Autodesk Fusion 360 part; units mm, degrees
(part 20 of 25)
sketch "Top Component Outlines" plane through (0, 0, 0) normal (0, 0, 1) x (1, 0, 0)
  arc A0 (71.501, 48.2981) -> (71.501, 48.2219) centre (71.501, 48.26) ccw
  arc A1 (71.501, 48.2219) -> (71.501, 48.2981) centre (71.501, 48.26) ccw
  arc A2 (76.0349, 48.514) -> (76.1111, 48.514) centre (76.073, 48.514) ccw
  arc A3 (73.9775, 50.292) -> (73.8505, 50.292) centre (73.914, 50.292) ccw
  arc A4 (75.819, 48.2219) -> (75.819, 48.2981) centre (75.819, 48.26) ccw
  arc A5 (73.9775, 49.53) -> (73.8505, 49.53) centre (73.914, 49.53) ccw
  arc A6 (71.501, 50.8) -> (71.247, 50.546) centre (71.501, 50.546) ccw
  arc A7 (76.1111, 50.546) -> (76.0349, 50.546) centre (76.073, 50.546) ccw
  arc A8 (71.501, 50.7619) -> (71.501, 50.8381) centre (71.501, 50.8) ccw
  arc A9 (73.3425, 49.53) -> (73.4695, 49.53) centre (73.406, 49.53) ccw
  arc A10 (71.501, 50.8381) -> (71.501, 50.7619) centre (71.501, 50.8) ccw
  arc A11 (71.2851, 48.514) -> (71.2089, 48.514) centre (71.247, 48.514) ccw
  arc A12 (73.3425, 48.768) -> (73.4695, 48.768) centre (73.406, 48.768) ccw
  line L0 (74.041, 49.53) -> (73.914, 49.53)
  line L1 (71.247, 50.546) -> (71.247, 48.514)
  arc A13 (71.2089, 48.514) -> (71.2851, 48.514) centre (71.247, 48.514) ccw
  line L2 (71.501, 50.8) -> (75.819, 50.8)
  arc A14 (76.0349, 50.546) -> (76.1111, 50.546) centre (76.073, 50.546) ccw
  arc A15 (76.1111, 48.514) -> (76.0349, 48.514) centre (76.073, 48.514) ccw
  arc A16 (71.2089, 50.546) -> (71.2851, 50.546) centre (71.247, 50.546) ccw
  line L3 (73.914, 49.53) -> (73.914, 48.768)
  line L4 (75.819, 48.26) -> (71.501, 48.26)
  arc A17 (71.247, 48.514) -> (71.501, 48.26) centre (71.501, 48.514) ccw
  arc A18 (73.4695, 50.292) -> (73.3425, 50.292) centre (73.406, 50.292) ccw
  arc A19 (75.819, 50.8381) -> (75.819, 50.7619) centre (75.819, 50.8) ccw
  arc A20 (73.914, 49.5681) -> (73.914, 49.4919) centre (73.914, 49.53) ccw
  arc A21 (74.041, 49.4919) -> (74.041, 49.5681) centre (74.041, 49.53) ccw
  arc A22 (76.073, 50.546) -> (75.819, 50.8) centre (75.819, 50.546) ccw
  arc A23 (75.819, 50.7619) -> (75.819, 50.8381) centre (75.819, 50.8) ccw
  arc A24 (71.2851, 50.546) -> (71.2089, 50.546) centre (71.247, 50.546) ccw
  arc A25 (75.819, 48.26) -> (76.073, 48.514) centre (75.819, 48.514) ccw
  arc A26 (75.819, 48.2981) -> (75.819, 48.2219) centre (75.819, 48.26) ccw
  line L5 (73.406, 49.53) -> (73.279, 49.53)
  arc A27 (73.406, 49.4919) -> (73.406, 49.5681) centre (73.406, 49.53) ccw
  arc A28 (73.8505, 49.53) -> (73.9775, 49.53) centre (73.914, 49.53) ccw
  arc A29 (73.4695, 49.53) -> (73.3425, 49.53) centre (73.406, 49.53) ccw
  arc A30 (73.279, 49.5681) -> (73.279, 49.4919) centre (73.279, 49.53) ccw
  line L6 (76.073, 50.546) -> (76.073, 48.514)
  arc A31 (73.8505, 48.768) -> (73.9775, 48.768) centre (73.914, 48.768) ccw
  line L7 (73.914, 49.53) -> (73.914, 50.292)
  line L8 (73.406, 50.292) -> (73.406, 49.53)
  line L9 (73.406, 49.53) -> (73.406, 48.768)
  arc A32 (14.605, 38.9509) -> (14.605, 39.0271) centre (14.605, 38.989) ccw
  line L10 (12.7, 37.338) -> (15.24, 37.338)
  line L11 (15.24, 37.338) -> (15.24, 37.846)
  line L12 (13.97, 38.989) -> (14.605, 38.989)
  arc A33 (13.97, 39.0271) -> (13.97, 38.9509) centre (13.97, 38.989) ccw
  arc A34 (15.2019, 36.957) -> (15.2781, 36.957) centre (15.24, 36.957) ccw
  arc A35 (50.3809, 18.669) -> (50.4571, 18.669) centre (50.419, 18.669) ccw
  line L13 (13.97, 38.354) -> (13.97, 38.989)
  arc A36 (14.605, 39.9669) -> (14.605, 40.0431) centre (14.605, 40.005) ccw
  line L14 (14.351, 41.021) -> (14.351, 42.926)
  arc A37 (50.4571, 19.05) -> (50.3809, 19.05) centre (50.419, 19.05) ccw
  arc A38 (52.07, 20.574) -> (52.07, 14.986) centre (52.07, 17.78) ccw
  arc A39 (15.2781, 41.021) -> (15.2019, 41.021) centre (15.24, 41.021) ccw
  line L15 (13.589, 36.957) -> (13.589, 35.052)
  arc A40 (15.24, 36.9189) -> (15.24, 36.9951) centre (15.24, 36.957) ccw
  line L16 (13.589, 35.052) -> (14.351, 35.052)
  arc A41 (52.07, 14.986) -> (52.07, 20.574) centre (52.07, 17.78) ccw
  line L17 (14.351, 42.926) -> (13.589, 42.926)
  line L18 (50.419, 19.05) -> (50.419, 19.431)
  line L19 (13.335, 40.005) -> (14.605, 40.005)
  arc A42 (13.9319, 38.354) -> (14.0081, 38.354) centre (13.97, 38.354) ccw
  line L20 (15.24, 37.846) -> (12.7, 37.846)
  arc A43 (14.0081, 38.989) -> (13.9319, 38.989) centre (13.97, 38.989) ccw
  line L21 (13.335, 38.989) -> (13.97, 38.989)
  arc A44 (12.7, 41.0591) -> (12.7, 40.9829) centre (12.7, 41.021) ccw
  line L22 (13.589, 41.021) -> (14.351, 41.021)
  line L23 (14.605, 40.005) -> (13.97, 38.989)
  arc A45 (50.4571, 19.431) -> (50.3809, 19.431) centre (50.419, 19.431) ccw
  arc A46 (50.038, 19.0881) -> (50.038, 19.0119) centre (50.038, 19.05) ccw
  line L24 (13.97, 38.989) -> (13.335, 40.005)
  arc A47 (15.24, 40.9829) -> (15.24, 41.0591) centre (15.24, 41.021) ccw
  line L25 (15.24, 41.021) -> (15.24, 36.957)
  line L26 (50.419, 18.669) -> (50.419, 19.05)
  arc A48 (12.7381, 41.021) -> (12.6619, 41.021) centre (12.7, 41.021) ccw
  arc A49 (13.9377, 39.0092) -> (14.0023, 38.9688) centre (13.97, 38.989) ccw
  arc A50 (12.7, 36.9951) -> (12.7, 36.9189) centre (12.7, 36.957) ccw
  arc A51 (14.0081, 40.513) -> (13.9319, 40.513) centre (13.97, 40.513) ccw
  arc A52 (13.3673, 40.0252) -> (13.3027, 39.9848) centre (13.335, 40.005) ccw
  arc A53 (13.9377, 38.9688) -> (14.0023, 39.0092) centre (13.97, 38.989) ccw
  arc A54 (13.335, 39.0271) -> (13.335, 38.9509) centre (13.335, 38.989) ccw
  line L27 (13.589, 42.926) -> (13.589, 41.021)
  line L28 (13.97, 38.989) -> (13.97, 40.513)
  arc A55 (13.97, 38.9509) -> (13.97, 39.0271) centre (13.97, 38.989) ccw
  line L29 (12.7, 37.846) -> (12.7, 37.338)
  arc A56 (50.419, 19.0119) -> (50.419, 19.0881) centre (50.419, 19.05) ccw
  line L30 (12.7, 36.957) -> (12.7, 41.021)
  arc A57 (13.9319, 38.989) -> (14.0081, 38.989) centre (13.97, 38.989) ccw
  arc A58 (14.6373, 39.9848) -> (14.5727, 40.0252) centre (14.605, 40.005) ccw
  arc A59 (13.335, 40.0431) -> (13.335, 39.9669) centre (13.335, 40.005) ccw
  arc A60 (25.3492, 24.765) -> (25.4508, 24.765) centre (25.4, 24.765) ccw
  arc A61 (50.8, 19.0119) -> (50.8, 19.0881) centre (50.8, 19.05) ccw
  line L31 (12.7, 36.957) -> (15.24, 36.957)
  line L32 (25.4, 26.035) -> (25.4, 24.765)
  arc A62 (50.3809, 19.05) -> (50.4571, 19.05) centre (50.419, 19.05) ccw
  arc A63 (12.6619, 36.957) -> (12.7381, 36.957) centre (12.7, 36.957) ccw
  arc A64 (50.419, 19.0881) -> (50.419, 19.0119) centre (50.419, 19.05) ccw
  line L33 (14.351, 36.957) -> (13.589, 36.957)
  line L34 (15.24, 41.021) -> (12.7, 41.021)
  line L35 (14.351, 35.052) -> (14.351, 36.957)
  line L36 (50.038, 19.05) -> (50.419, 19.05)
  line L37 (50.419, 19.05) -> (50.8, 19.05)
  line L38 (72.39, 45.085) -> (72.39, 43.815)
  arc A65 (72.3392, 43.815) -> (72.4408, 43.815) centre (72.39, 43.815) ccw
  arc A66 (25.4508, 26.035) -> (25.3492, 26.035) centre (25.4, 26.035) ccw
  arc A67 (72.4408, 45.085) -> (72.3392, 45.085) centre (72.39, 45.085) ccw
  line L39 (38.1, 26.035) -> (38.1, 24.765)
  arc A68 (82.6008, 32.385) -> (82.4992, 32.385) centre (82.55, 32.385) ccw
  line L40 (82.55, 32.385) -> (82.55, 31.115)
  arc A69 (82.4992, 31.115) -> (82.6008, 31.115) centre (82.55, 31.115) ccw
  arc A70 (38.1508, 26.035) -> (38.0492, 26.035) centre (38.1, 26.035) ccw
  arc A71 (67.3608, 43.815) -> (67.2592, 43.815) centre (67.31, 43.815) ccw
  line L41 (57.15, 43.815) -> (57.15, 42.545)
  line L42 (59.69, 31.115) -> (59.69, 32.385)
  arc A72 (22.9108, 50.165) -> (22.8092, 50.165) centre (22.86, 50.165) ccw
  arc A73 (22.8092, 48.895) -> (22.9108, 48.895) centre (22.86, 48.895) ccw
  arc A74 (57.2008, 43.815) -> (57.0992, 43.815) centre (57.15, 43.815) ccw
  arc A75 (33.0962, 37.9476) -> (33.0962, 38.2524) centre (33.0962, 38.1) ccw
  arc A76 (72.4408, 32.385) -> (72.3392, 32.385) centre (72.39, 32.385) ccw
  arc A77 (59.7408, 32.385) -> (59.6392, 32.385) centre (59.69, 32.385) ccw
  arc A78 (67.2592, 42.545) -> (67.3608, 42.545) centre (67.31, 42.545) ccw
  arc A79 (27.8638, 38.2524) -> (27.8638, 37.9476) centre (27.8638, 38.1) ccw
  line L43 (33.0962, 38.1) -> (27.8638, 38.1)
  arc A80 (72.3392, 31.115) -> (72.4408, 31.115) centre (72.39, 31.115) ccw
  arc A81 (67.3608, 32.385) -> (67.2592, 32.385) centre (67.31, 32.385) ccw
  arc A82 (67.2592, 31.115) -> (67.3608, 31.115) centre (67.31, 31.115) ccw
  arc A83 (59.6392, 31.115) -> (59.7408, 31.115) centre (59.69, 31.115) ccw
  line L44 (22.86, 48.895) -> (22.86, 50.165)
  arc A84 (33.0962, 34.1376) -> (33.0962, 34.4424) centre (33.0962, 34.29) ccw
  line L45 (72.39, 32.385) -> (72.39, 31.115)
  arc A85 (57.0992, 42.545) -> (57.2008, 42.545) centre (57.15, 42.545) ccw
  line L46 (33.0962, 34.29) -> (27.8638, 34.29)
  arc A86 (46.9392, 24.765) -> (47.0408, 24.765) centre (46.99, 24.765) ccw
  line L47 (54.61, 26.035) -> (54.61, 24.765)
  arc A87 (54.5592, 24.765) -> (54.6608, 24.765) centre (54.61, 24.765) ccw
  arc A88 (82.4992, 43.815) -> (82.6008, 43.815) centre (82.55, 43.815) ccw
  arc A89 (38.0492, 24.765) -> (38.1508, 24.765) centre (38.1, 24.765) ccw
  arc A90 (82.6008, 45.085) -> (82.4992, 45.085) centre (82.55, 45.085) ccw
  arc A91 (10.1092, 48.895) -> (10.2108, 48.895) centre (10.16, 48.895) ccw
  arc A92 (27.8638, 34.4424) -> (27.8638, 34.1376) centre (27.8638, 34.29) ccw
  line L48 (82.55, 45.085) -> (82.55, 43.815)
  line L49 (10.16, 48.895) -> (10.16, 50.165)
  line L50 (67.31, 31.115) -> (67.31, 32.385)
  arc A93 (10.2108, 50.165) -> (10.1092, 50.165) centre (10.16, 50.165) ccw
  line L51 (67.31, 43.815) -> (67.31, 42.545)
  line L52 (34.925, 15.24) -> (34.29, 15.875)
  arc A94 (36.8659, 15.8391) -> (36.7941, 15.9109) centre (36.83, 15.875) ccw
  arc A95 (34.2541, 17.1809) -> (34.3259, 17.1091) centre (34.29, 17.145) ccw
  arc A96 (38.6991, 15.2759) -> (38.7709, 15.2041) centre (38.735, 15.24) ccw
  arc A97 (39.4059, 15.8391) -> (39.3341, 15.9109) centre (39.37, 15.875) ccw
  line L53 (36.195, 15.24) -> (34.925, 15.24)
  line L54 (29.845, 17.78) -> (31.115, 17.78)
  arc A98 (29.8809, 17.7441) -> (29.8091, 17.8159) centre (29.845, 17.78) ccw
  line L55 (26.67, 17.145) -> (27.305, 17.78)
  line L56 (46.99, 26.035) -> (46.99, 24.765)
  line L57 (37.465, 17.78) -> (36.83, 17.145)
  arc A99 (31.0791, 15.2759) -> (31.1509, 15.2041) centre (31.115, 15.24) ccw
  arc A100 (37.5009, 17.7441) -> (37.4291, 17.8159) centre (37.465, 17.78) ccw
  line L58 (34.925, 17.78) -> (36.195, 17.78)
  line L59 (31.115, 17.78) -> (31.75, 17.145)
  arc A101 (31.1509, 17.8159) -> (31.0791, 17.7441) centre (31.115, 17.78) ccw
  arc A102 (39.3341, 17.1091) -> (39.4059, 17.1809) centre (39.37, 17.145) ccw
  line L60 (36.83, 15.875) -> (36.195, 15.24)
  arc A103 (36.2309, 17.8159) -> (36.1591, 17.7441) centre (36.195, 17.78) ccw
  arc A104 (36.7941, 17.1091) -> (36.8659, 17.1809) centre (36.83, 17.145) ccw
  arc A105 (34.925, 15.2908) -> (34.925, 15.1892) centre (34.925, 15.24) ccw
  arc A106 (36.195, 15.1892) -> (36.195, 15.2908) centre (36.195, 15.24) ccw
  arc A107 (36.7941, 17.1809) -> (36.8659, 17.1091) centre (36.83, 17.145) ccw
  arc A108 (37.465, 17.8308) -> (37.465, 17.7292) centre (37.465, 17.78) ccw
  arc A109 (38.735, 17.7292) -> (38.735, 17.8308) centre (38.735, 17.78) ccw
  line L61 (37.465, 17.78) -> (38.735, 17.78)
  arc A110 (38.7709, 17.8159) -> (38.6991, 17.7441) centre (38.735, 17.78) ccw
  arc A111 (36.195, 17.7292) -> (36.195, 17.8308) centre (36.195, 17.78) ccw
  line L62 (36.195, 17.78) -> (36.83, 17.145)
  arc A112 (34.8891, 15.2041) -> (34.9609, 15.2759) centre (34.925, 15.24) ccw
  arc A113 (34.925, 17.8308) -> (34.925, 17.7292) centre (34.925, 17.78) ccw
  line L63 (36.83, 15.875) -> (37.465, 15.24)
  arc A114 (31.115, 17.7292) -> (31.115, 17.8308) centre (31.115, 17.78) ccw
  arc A115 (54.6608, 26.035) -> (54.5592, 26.035) centre (54.61, 26.035) ccw
  arc A116 (47.0408, 26.035) -> (46.9392, 26.035) centre (46.99, 26.035) ccw
  line L64 (34.29, 17.145) -> (34.925, 17.78)
  arc A117 (36.1591, 15.2759) -> (36.2309, 15.2041) centre (36.195, 15.24) ccw
  arc A118 (34.3259, 15.9109) -> (34.2541, 15.8391) centre (34.29, 15.875) ccw
  arc A119 (38.735, 15.1892) -> (38.735, 15.2908) centre (38.735, 15.24) ccw
  arc A120 (34.9609, 17.7441) -> (34.8891, 17.8159) centre (34.925, 17.78) ccw
  arc A121 (29.845, 17.8308) -> (29.845, 17.7292) centre (29.845, 17.78) ccw
  arc A122 (37.4291, 15.2041) -> (37.5009, 15.2759) centre (37.465, 15.24) ccw
  arc A123 (36.8659, 15.9109) -> (36.7941, 15.8391) centre (36.83, 15.875) ccw
  line L65 (31.75, 15.875) -> (31.115, 15.24)
  line L66 (38.735, 17.78) -> (39.37, 17.145)
  arc A124 (37.465, 15.2908) -> (37.465, 15.1892) centre (37.465, 15.24) ccw
  arc A125 (31.7141, 17.1091) -> (31.7859, 17.1809) centre (31.75, 17.145) ccw
  line L67 (38.735, 15.24) -> (37.465, 15.24)
  line L68 (39.37, 15.875) -> (38.735, 15.24)
  line L69 (31.75, 17.145) -> (32.385, 17.78)
  arc A126 (27.2691, 15.2041) -> (27.3409, 15.2759) centre (27.305, 15.24) ccw
  arc A127 (29.845, 15.2908) -> (29.845, 15.1892) centre (29.845, 15.24) ccw
  line L70 (24.13, 17.145) -> (24.765, 17.78)
  line L71 (26.035, 17.78) -> (26.67, 17.145)
  arc A128 (33.6191, 15.2759) -> (33.6909, 15.2041) centre (33.655, 15.24) ccw
  arc A129 (28.575, 15.1892) -> (28.575, 15.2908) centre (28.575, 15.24) ccw
  line L72 (34.29, 15.875) -> (33.655, 15.24)
  line L73 (32.385, 17.78) -> (33.655, 17.78)
  line L74 (24.765, 17.78) -> (26.035, 17.78)
  arc A130 (32.3491, 15.2041) -> (32.4209, 15.2759) centre (32.385, 15.24) ccw
  arc A131 (27.305, 15.2908) -> (27.305, 15.1892) centre (27.305, 15.24) ccw
  arc A132 (27.305, 17.8308) -> (27.305, 17.7292) centre (27.305, 17.78) ccw
  line L75 (29.845, 17.78) -> (29.21, 17.145)
  line L76 (24.13, 15.875) -> (23.495, 15.24)
  arc A133 (22.225, 17.8308) -> (22.225, 17.7292) centre (22.225, 17.78) ccw
  arc A134 (24.0941, 17.1091) -> (24.1659, 17.1809) centre (24.13, 17.145) ccw
  arc A135 (29.2459, 15.9109) -> (29.1741, 15.8391) centre (29.21, 15.875) ccw
  arc A136 (24.1659, 15.8391) -> (24.0941, 15.9109) centre (24.13, 15.875) ccw
  arc A137 (24.8009, 17.7441) -> (24.7291, 17.8159) centre (24.765, 17.78) ccw
  arc A138 (32.385, 17.8308) -> (32.385, 17.7292) centre (32.385, 17.78) ccw
  line L77 (33.655, 17.78) -> (34.29, 17.145)
  arc A139 (34.3259, 15.8391) -> (34.2541, 15.9109) centre (34.29, 15.875) ccw
  arc A140 (31.7859, 15.9109) -> (31.7141, 15.8391) centre (31.75, 15.875) ccw
  line L78 (32.385, 15.24) -> (31.75, 15.875)
  arc A141 (26.035, 17.7292) -> (26.035, 17.8308) centre (26.035, 17.78) ccw
  arc A142 (34.2541, 17.1091) -> (34.3259, 17.1809) centre (34.29, 17.145) ccw
  line L79 (31.115, 15.24) -> (29.845, 15.24)
  arc A143 (32.4209, 17.7441) -> (32.3491, 17.8159) centre (32.385, 17.78) ccw
  arc A144 (27.3409, 17.7441) -> (27.2691, 17.8159) centre (27.305, 17.78) ccw
  arc A145 (26.7059, 15.9109) -> (26.6341, 15.8391) centre (26.67, 15.875) ccw
  arc A146 (23.5309, 17.8159) -> (23.4591, 17.7441) centre (23.495, 17.78) ccw
  line L80 (28.575, 15.24) -> (27.305, 15.24)
  arc A147 (41.8741, 17.1091) -> (41.9459, 17.1809) centre (41.91, 17.145) ccw
  arc A148 (24.0941, 17.1809) -> (24.1659, 17.1091) centre (24.13, 17.145) ccw
  line L81 (27.305, 17.78) -> (28.575, 17.78)
  arc A149 (31.115, 15.1892) -> (31.115, 15.2908) centre (31.115, 15.24) ccw
  arc A150 (29.1741, 17.1091) -> (29.2459, 17.1809) centre (29.21, 17.145) ccw
  arc A151 (32.385, 15.2908) -> (32.385, 15.1892) centre (32.385, 15.24) ccw
  arc A152 (26.6341, 17.1809) -> (26.7059, 17.1091) centre (26.67, 17.145) ccw
  arc A153 (28.5391, 15.2759) -> (28.6109, 15.2041) centre (28.575, 15.24) ccw
  arc A154 (26.6341, 17.1091) -> (26.7059, 17.1809) centre (26.67, 17.145) ccw
  line L82 (23.495, 17.78) -> (24.13, 17.145)
  arc A155 (28.6109, 17.8159) -> (28.5391, 17.7441) centre (28.575, 17.78) ccw
  arc A156 (21.5541, 17.1809) -> (21.6259, 17.1091) centre (21.59, 17.145) ccw
  line L83 (28.575, 17.78) -> (29.21, 17.145)
  line L84 (29.21, 15.875) -> (28.575, 15.24)
  line L85 (29.21, 15.875) -> (29.845, 15.24)
  arc A157 (29.1741, 17.1809) -> (29.2459, 17.1091) centre (29.21, 17.145) ccw
  arc A158 (31.7859, 15.8391) -> (31.7141, 15.9109) centre (31.75, 15.875) ccw
  arc A159 (23.4591, 15.2759) -> (23.5309, 15.2041) centre (23.495, 15.24) ccw
  arc A160 (29.2459, 15.8391) -> (29.1741, 15.9109) centre (29.21, 15.875) ccw
  arc A161 (28.575, 17.7292) -> (28.575, 17.8308) centre (28.575, 17.78) ccw
  arc A162 (23.495, 17.7292) -> (23.495, 17.8308) centre (23.495, 17.78) ccw
  line L86 (22.225, 17.78) -> (23.495, 17.78)
  arc A163 (31.7141, 17.1809) -> (31.7859, 17.1091) centre (31.75, 17.145) ccw
  arc A164 (33.6909, 17.8159) -> (33.6191, 17.7441) centre (33.655, 17.78) ccw
  arc A165 (29.8091, 15.2041) -> (29.8809, 15.2759) centre (29.845, 15.24) ccw
  line L87 (33.655, 15.24) -> (32.385, 15.24)
  arc A166 (26.0709, 17.8159) -> (25.9991, 17.7441) centre (26.035, 17.78) ccw
  arc A167 (33.655, 15.1892) -> (33.655, 15.2908) centre (33.655, 15.24) ccw
  arc A168 (24.765, 17.8308) -> (24.765, 17.7292) centre (24.765, 17.78) ccw
  line L88 (27.305, 15.24) -> (26.67, 15.875)
  arc A169 (33.655, 17.7292) -> (33.655, 17.8308) centre (33.655, 17.78) ccw
  line L89 (26.035, 15.24) -> (24.765, 15.24)
  arc A170 (21.6259, 15.9109) -> (21.5541, 15.8391) centre (21.59, 15.875) ccw
  arc A171 (3.5433, 5.0673) -> (4.1317, 3.8643) centre (5.067, 5.0672) ccw
  arc A172 (40.005, 17.8308) -> (40.005, 17.7292) centre (40.005, 17.78) ccw
  arc A173 (6.5913, 5.0673) -> (5.9817, 6.2865) centre (5.0675, 5.0674) ccw
  arc A174 (3.0353, 5.0673) -> (3.7547, 3.5161) centre (5.0674, 5.0673) ccw
  arc A175 (6.3881, 7.3342) -> (6.3881, 7.2708) centre (6.3881, 7.3025) ccw
  arc A176 (26.7059, 15.8391) -> (26.6341, 15.9109) centre (26.67, 15.875) ccw
  arc A177 (4.0591, 6.8316) -> (3.0353, 5.0673) centre (5.0676, 5.0672) ccw
  arc A178 (41.8592, 15.875) -> (41.9608, 15.875) centre (41.91, 15.875) ccw
  arc A179 (7.1755, 7.2708) -> (7.1755, 7.3342) centre (7.1755, 7.3025) ccw
  arc A180 (6.3682, 3.5063) -> (7.0993, 5.0673) centre (5.0675, 5.0672) ccw
  arc A181 (41.275, 17.7292) -> (41.275, 17.8308) centre (41.275, 17.78) ccw
  arc A182 (21.5392, 15.875) -> (21.6408, 15.875) centre (21.59, 15.875) ccw
  line L90 (22.225, 17.78) -> (21.59, 17.145)
  arc A183 (9.098, 33.2692) -> (9.098, 33.3708) centre (9.098, 33.32) ccw
  arc A184 (1.9872, 33.32) -> (2.0888, 33.32) centre (2.038, 33.32) ccw
  line L91 (23.495, 15.24) -> (22.225, 15.24)
  line L92 (2.038, 45.42) -> (9.098, 45.42)
  arc A185 (24.7291, 15.2041) -> (24.8009, 15.2759) centre (24.765, 15.24) ccw
  arc A186 (41.275, 15.1892) -> (41.275, 15.2908) centre (41.275, 15.24) ccw
  arc A187 (26.035, 15.1892) -> (26.035, 15.2908) centre (26.035, 15.24) ccw
  arc A188 (25.9991, 15.2759) -> (26.0709, 15.2041) centre (26.035, 15.24) ccw
  arc A189 (21.6408, 17.145) -> (21.5392, 17.145) centre (21.59, 17.145) ccw
  line L93 (21.59, 15.875) -> (22.225, 15.24)
  arc A190 (41.3109, 17.8159) -> (41.2391, 17.7441) centre (41.275, 17.78) ccw
  line L94 (41.275, 15.24) -> (40.005, 15.24)
  line L95 (41.91, 15.875) -> (41.275, 15.24)
  arc A191 (39.9691, 15.2041) -> (40.0409, 15.2759) centre (40.005, 15.24) ccw
  arc A192 (23.495, 15.1892) -> (23.495, 15.2908) centre (23.495, 15.24) ccw
  line L96 (21.59, 17.145) -> (21.59, 15.875)
  arc A193 (24.765, 15.2908) -> (24.765, 15.1892) centre (24.765, 15.24) ccw
  line L97 (9.098, 33.32) -> (9.098, 45.42)
  arc A194 (22.225, 15.2908) -> (22.225, 15.1892) centre (22.225, 15.24) ccw
  arc A195 (41.2391, 15.2759) -> (41.3109, 15.2041) centre (41.275, 15.24) ccw
  arc A196 (39.3341, 17.1809) -> (39.4059, 17.1091) centre (39.37, 17.145) ccw
  arc A197 (2.0888, 45.42) -> (1.9872, 45.42) centre (2.038, 45.42) ccw
  line L98 (24.765, 15.24) -> (24.13, 15.875)
  arc A198 (9.0472, 33.32) -> (9.1488, 33.32) centre (9.098, 33.32) ccw
  arc A199 (2.038, 33.3708) -> (2.038, 33.2692) centre (2.038, 33.32) ccw
  arc A200 (9.098, 45.3692) -> (9.098, 45.4708) centre (9.098, 45.42) ccw
  arc A201 (41.9608, 17.145) -> (41.8592, 17.145) centre (41.91, 17.145) ccw
  arc A202 (40.0409, 17.7441) -> (39.9691, 17.8159) centre (40.005, 17.78) ccw
  line L99 (2.038, 45.42) -> (2.038, 33.32)
  line L100 (40.005, 17.78) -> (39.37, 17.145)
  arc A203 (40.005, 15.2908) -> (40.005, 15.1892) centre (40.005, 15.24) ccw
  arc A204 (39.4059, 15.9109) -> (39.3341, 15.8391) centre (39.37, 15.875) ccw
  line L101 (40.005, 17.78) -> (41.275, 17.78)
  arc A205 (2.038, 45.4708) -> (2.038, 45.3692) centre (2.038, 45.42) ccw
  line L102 (6.7945, 7.6581) -> (6.7945, 6.9215)
  line L103 (41.275, 17.78) -> (41.91, 17.145)
  arc A206 (22.1891, 15.2041) -> (22.2609, 15.2759) centre (22.225, 15.24) ccw
  line L104 (41.91, 17.145) -> (41.91, 15.875)
  line L105 (9.098, 33.32) -> (2.038, 33.32)
  arc A207 (6.7628, 6.9215) -> (6.8262, 6.9215) centre (6.7945, 6.9215) ccw
  arc A208 (6.8262, 7.6581) -> (6.7628, 7.6581) centre (6.7945, 7.6581) ccw
  line L106 (26.67, 15.875) -> (26.035, 15.24)
  arc A209 (41.9459, 15.8391) -> (41.8741, 15.9109) centre (41.91, 15.875) ccw
  arc A210 (9.1488, 45.42) -> (9.0472, 45.42) centre (9.098, 45.42) ccw
  arc A211 (7.0993, 5.0673) -> (6.0235, 6.8602) centre (5.0674, 5.0673) ccw
  line L107 (39.37, 15.875) -> (40.005, 15.24)
  arc A212 (22.2609, 17.7441) -> (22.1891, 17.8159) centre (22.225, 17.78) ccw
  line L108 (6.3881, 7.3025) -> (7.1755, 7.3025)
  arc A213 (24.1659, 15.9109) -> (24.0941, 15.8391) centre (24.13, 15.875) ccw
  arc A214 (74.676, 13.5509) -> (74.676, 13.6271) centre (74.676, 13.589) ccw
  line L109 (80.772, 11.557) -> (80.772, 13.335)
  arc A215 (75.1571, 13.4351) -> (75.2109, 13.4889) centre (75.184, 13.462) ccw
  line L110 (80.01, 11.43) -> (80.137, 11.303)
  arc A216 (75.184, 13.5001) -> (75.184, 13.4239) centre (75.184, 13.462) ccw
  arc A217 (74.676, 11.2649) -> (74.676, 11.3411) centre (74.676, 11.303) ccw
  arc A218 (74.676, 13.589) -> (74.422, 13.335) centre (74.676, 13.335) ccw
  line L111 (74.676, 13.589) -> (75.057, 13.589)
  line L112 (81.6356, 12.1412) -> (81.6356, 12.7508)
  arc A219 (80.518, 11.2649) -> (80.518, 11.3411) centre (80.518, 11.303) ccw
  arc A220 (14.8558, 3.8399) -> (15.494, 5.08) centre (13.97, 5.0801) ccw
  arc A221 (80.518, 13.6271) -> (80.518, 13.5509) centre (80.518, 13.589) ccw
  arc A222 (13.0344, 6.283) -> (12.446, 5.08) centre (13.9697, 5.0801) ccw
  arc A223 (15.2908, 7.3469) -> (15.2908, 7.2835) centre (15.2908, 7.3152) ccw
  line L113 (15.6972, 7.6708) -> (15.6972, 6.9342)
  arc A224 (74.3839, 13.335) -> (74.4601, 13.335) centre (74.422, 13.335) ccw
  arc A225 (80.518, 11.3411) -> (80.518, 11.2649) centre (80.518, 11.303) ccw
  arc A226 (11.938, 5.08) -> (12.6574, 3.5288) centre (13.9701, 5.08) ccw
  arc A227 (15.6654, 6.9342) -> (15.729, 6.9342) centre (15.6972, 6.9342) ccw
  arc A228 (5.9531, 3.8272) -> (6.5913, 5.0673) centre (5.0673, 5.0674) ccw
  arc A229 (15.729, 7.6708) -> (15.6654, 7.6708) centre (15.6972, 7.6708) ccw
  arc A230 (80.7339, 11.557) -> (80.8101, 11.557) centre (80.772, 11.557) ccw
  arc A231 (75.0301, 11.3299) -> (75.0839, 11.2761) centre (75.057, 11.303) ccw
  arc A232 (15.494, 5.08) -> (14.8844, 6.2992) centre (13.9702, 5.0801) ccw
  arc A233 (12.9618, 6.8443) -> (11.938, 5.08) centre (13.9703, 5.0799) ccw
  arc A234 (80.01, 11.3919) -> (80.01, 11.4681) centre (80.01, 11.43) ccw
  arc A235 (74.422, 11.557) -> (74.676, 11.303) centre (74.676, 11.557) ccw
  line L114 (80.772, 12.1412) -> (81.6356, 12.1412)
  line L115 (81.6356, 12.7508) -> (80.772, 12.7508)
  line L116 (80.518, 11.303) -> (80.137, 11.303)
  arc A236 (75.057, 11.2649) -> (75.057, 11.3411) centre (75.057, 11.303) ccw
  arc A237 (74.676, 11.3411) -> (74.676, 11.2649) centre (74.676, 11.303) ccw
  arc A238 (12.446, 5.08) -> (13.0344, 3.877) centre (13.9697, 5.0799) ccw
  line L117 (15.2908, 7.3152) -> (16.0782, 7.3152)
  arc A239 (80.518, 11.303) -> (80.772, 11.557) centre (80.518, 11.557) ccw
  arc A240 (74.3839, 11.557) -> (74.4601, 11.557) centre (74.422, 11.557) ccw
  arc A241 (80.1639, 13.5621) -> (80.1101, 13.6159) centre (80.137, 13.589) ccw
  arc A242 (4.1317, 6.2703) -> (3.5433, 5.0673) centre (5.067, 5.0674) ccw
  arc A243 (80.1101, 11.2761) -> (80.1639, 11.3299) centre (80.137, 11.303) ccw
  arc A244 (80.772, 13.335) -> (80.518, 13.589) centre (80.518, 13.335) ccw
  arc A245 (80.137, 13.6271) -> (80.137, 13.5509) centre (80.137, 13.589) ccw
  arc A246 (16.002, 5.08) -> (14.9262, 6.8729) centre (13.9701, 5.08) ccw
  arc A247 (15.2709, 3.519) -> (16.002, 5.08) centre (13.9702, 5.0799) ccw
  line L118 (73.5584, 12.7508) -> (73.5584, 12.1412)
  line L119 (80.01, 11.43) -> (75.184, 11.43)
  line L120 (75.184, 13.462) -> (75.057, 13.589)
  line L121 (74.676, 11.303) -> (75.057, 11.303)
  arc A248 (74.676, 13.6271) -> (74.676, 13.5509) centre (74.676, 13.589) ccw
  arc A249 (79.9831, 13.4889) -> (80.0369, 13.4351) centre (80.01, 13.462) ccw
  arc A250 (74.4601, 11.557) -> (74.3839, 11.557) centre (74.422, 11.557) ccw
  arc A251 (75.0839, 13.6159) -> (75.0301, 13.5621) centre (75.057, 13.589) ccw
  line L122 (80.772, 12.7508) -> (80.772, 12.1412)
  arc A252 (16.0782, 7.2835) -> (16.0782, 7.3469) centre (16.0782, 7.3152) ccw
  arc A253 (75.2109, 11.4031) -> (75.1571, 11.4569) centre (75.184, 11.43) ccw
  arc A254 (80.0369, 11.4569) -> (79.9831, 11.4031) centre (80.01, 11.43) ccw
  arc A255 (80.7339, 13.335) -> (80.8101, 13.335) centre (80.772, 13.335) ccw
  line L123 (74.422, 12.7508) -> (73.5584, 12.7508)
  arc A256 (80.8101, 11.557) -> (80.7339, 11.557) centre (80.772, 11.557) ccw
  arc A257 (80.137, 11.3411) -> (80.137, 11.2649) centre (80.137, 11.303) ccw
  arc A258 (75.184, 11.4681) -> (75.184, 11.3919) centre (75.184, 11.43) ccw
  line L124 (75.184, 11.43) -> (75.057, 11.303)
  line L125 (80.01, 13.462) -> (80.137, 13.589)
  line L126 (80.01, 13.462) -> (75.184, 13.462)
  arc A259 (75.057, 13.5509) -> (75.057, 13.6271) centre (75.057, 13.589) ccw
  line L127 (73.5584, 12.1412) -> (74.422, 12.1412)
  arc A260 (13.1064, 10.3124) -> (13.1064, 10.2362) centre (13.1064, 10.2743) ccw
  arc A261 (7.2644, 12.5603) -> (7.0104, 12.3063) centre (7.2644, 12.3063) ccw
  arc A262 (7.6185, 10.3012) -> (7.6723, 10.2474) centre (7.6454, 10.2743) ccw
  line L128 (14.224, 11.1125) -> (14.224, 11.7221)
  line L129 (74.422, 12.1412) -> (74.422, 12.7508)
  arc A263 (7.7724, 10.4394) -> (7.7724, 10.3632) centre (7.7724, 10.4013) ccw
  arc A264 (12.7523, 12.5334) -> (12.6985, 12.5872) centre (12.7254, 12.5603) ccw
  arc A265 (13.1064, 10.2362) -> (13.1064, 10.3124) centre (13.1064, 10.2743) ccw
  line L130 (12.5984, 10.4013) -> (12.7254, 10.2743)
  arc A266 (13.1064, 12.5984) -> (13.1064, 12.5222) centre (13.1064, 12.5603) ccw
  line L131 (80.518, 13.589) -> (80.137, 13.589)
  arc A267 (13.3223, 12.3063) -> (13.3985, 12.3063) centre (13.3604, 12.3063) ccw
  arc A268 (12.5984, 10.3632) -> (12.5984, 10.4394) centre (12.5984, 10.4013) ccw
  arc A269 (12.5715, 12.4602) -> (12.6253, 12.4064) centre (12.5984, 12.4333) ccw
  line L132 (7.0104, 12.3063) -> (7.0104, 10.5283)
  arc A270 (12.6985, 10.2474) -> (12.7523, 10.3012) centre (12.7254, 10.2743) ccw
  line L133 (7.7724, 10.4013) -> (12.5984, 10.4013)
  arc A271 (7.7455, 12.4064) -> (7.7993, 12.4602) centre (7.7724, 12.4333) ccw
  arc A272 (12.7254, 12.5984) -> (12.7254, 12.5222) centre (12.7254, 12.5603) ccw
  arc A273 (7.2644, 12.5984) -> (7.2644, 12.5222) centre (7.2644, 12.5603) ccw
  line L134 (13.3604, 12.3063) -> (13.3604, 10.5283)
  line L135 (7.7724, 10.4013) -> (7.6454, 10.2743)
  arc A274 (12.7254, 10.3124) -> (12.7254, 10.2362) centre (12.7254, 10.2743) ccw
  arc A275 (13.3223, 10.5283) -> (13.3985, 10.5283) centre (13.3604, 10.5283) ccw
  arc A276 (74.4601, 13.335) -> (74.3839, 13.335) centre (74.422, 13.335) ccw
  line L136 (14.224, 11.7221) -> (13.3604, 11.7221)
  arc A277 (7.2644, 10.3124) -> (7.2644, 10.2362) centre (7.2644, 10.2743) ccw
  arc A278 (13.1064, 10.2743) -> (13.3604, 10.5283) centre (13.1064, 10.5283) ccw
  arc A279 (7.7993, 10.3744) -> (7.7455, 10.4282) centre (7.7724, 10.4013) ccw
  arc A280 (7.0485, 10.5283) -> (6.9723, 10.5283) centre (7.0104, 10.5283) ccw
  arc A281 (7.2644, 12.5222) -> (7.2644, 12.5984) centre (7.2644, 12.5603) ccw
  arc A282 (13.3604, 12.3063) -> (13.1064, 12.5603) centre (13.1064, 12.3063) ccw
  line L137 (74.422, 11.557) -> (74.422, 13.335)
  arc A283 (7.6454, 10.2362) -> (7.6454, 10.3124) centre (7.6454, 10.2743) ccw
  arc A284 (7.6723, 12.5872) -> (7.6185, 12.5334) centre (7.6454, 12.5603) ccw
  line L138 (7.7724, 12.4333) -> (7.6454, 12.5603)
  line L139 (13.1064, 12.5603) -> (12.7254, 12.5603)
  arc A285 (7.6454, 12.5222) -> (7.6454, 12.5984) centre (7.6454, 12.5603) ccw
  line L140 (13.3604, 11.1125) -> (14.224, 11.1125)
  arc A286 (13.1064, 12.5222) -> (13.1064, 12.5984) centre (13.1064, 12.5603) ccw
  arc A287 (80.518, 13.5509) -> (80.518, 13.6271) centre (80.518, 13.589) ccw
  arc A288 (6.9723, 12.3063) -> (7.0485, 12.3063) centre (7.0104, 12.3063) ccw
  line L141 (7.2644, 10.2743) -> (7.6454, 10.2743)
  line L142 (13.3604, 11.7221) -> (13.3604, 11.1125)
  line L143 (6.1468, 11.1125) -> (7.0104, 11.1125)
  line L144 (6.1468, 11.7221) -> (6.1468, 11.1125)
  line L145 (7.0104, 11.1125) -> (7.0104, 11.7221)
  arc A289 (80.01, 13.4239) -> (80.01, 13.5001) centre (80.01, 13.462) ccw
  arc A290 (80.8101, 13.335) -> (80.7339, 13.335) centre (80.772, 13.335) ccw
  arc A291 (6.9723, 10.5283) -> (7.0485, 10.5283) centre (7.0104, 10.5283) ccw
  arc A292 (7.7724, 12.4714) -> (7.7724, 12.3952) centre (7.7724, 12.4333) ccw
  line L146 (7.7724, 12.4333) -> (12.5984, 12.4333)
  arc A293 (7.0104, 10.5283) -> (7.2644, 10.2743) centre (7.2644, 10.5283) ccw
  arc A294 (7.2644, 10.2362) -> (7.2644, 10.3124) centre (7.2644, 10.2743) ccw
  line L147 (7.0104, 11.7221) -> (6.1468, 11.7221)
  arc A295 (12.6253, 10.4282) -> (12.5715, 10.3744) centre (12.5984, 10.4013) ccw
  line L148 (7.2644, 12.5603) -> (7.6454, 12.5603)
  line L149 (13.1064, 10.2743) -> (12.7254, 10.2743)
  arc A296 (12.5984, 12.3952) -> (12.5984, 12.4714) centre (12.5984, 12.4333) ccw
  arc A297 (13.3985, 10.5283) -> (13.3223, 10.5283) centre (13.3604, 10.5283) ccw
  arc A298 (7.0485, 12.3063) -> (6.9723, 12.3063) centre (7.0104, 12.3063) ccw
  line L150 (12.5984, 12.4333) -> (12.7254, 12.5603)
  arc A299 (13.3985, 12.3063) -> (13.3223, 12.3063) centre (13.3604, 12.3063) ccw
  line L151 (81.5086, 25.0952) -> (81.5086, 25.7048)
  arc A300 (74.3331, 26.289) -> (74.2569, 26.289) centre (74.295, 26.289) ccw
  arc A301 (60.9869, 21.4899) -> (60.9331, 21.4361) centre (60.96, 21.463) ccw
  arc A302 (74.2569, 24.511) -> (74.3331, 24.511) centre (74.295, 24.511) ccw
  arc A303 (75.0301, 26.3891) -> (75.0839, 26.4429) centre (75.057, 26.416) ccw
  arc A304 (74.9569, 26.5699) -> (74.9031, 26.5161) centre (74.93, 26.543) ccw
  arc A305 (74.549, 26.5811) -> (74.549, 26.5049) centre (74.549, 26.543) ccw
  arc A306 (74.93, 24.2189) -> (74.93, 24.2951) centre (74.93, 24.257) ccw
  line L152 (75.057, 26.416) -> (74.93, 26.543)
  arc A307 (80.6069, 26.289) -> (80.6831, 26.289) centre (80.645, 26.289) ccw
  arc A308 (80.6831, 26.289) -> (80.6069, 26.289) centre (80.645, 26.289) ccw
  line L153 (73.4314, 25.7048) -> (73.4314, 25.0952)
  line L154 (80.645, 25.7048) -> (80.645, 25.0952)
  arc A309 (75.0839, 24.3571) -> (75.0301, 24.4109) centre (75.057, 24.384) ccw
  arc A310 (80.0369, 26.5161) -> (79.9831, 26.5699) centre (80.01, 26.543) ccw
  arc A311 (80.391, 26.5049) -> (80.391, 26.5811) centre (80.391, 26.543) ccw
  arc A312 (79.9831, 24.2301) -> (80.0369, 24.2839) centre (80.01, 24.257) ccw
  line L155 (80.391, 26.543) -> (80.01, 26.543)
  arc A313 (80.391, 26.5811) -> (80.391, 26.5049) centre (80.391, 26.543) ccw
  arc A314 (80.391, 24.2951) -> (80.391, 24.2189) centre (80.391, 24.257) ccw
  line L156 (75.057, 24.384) -> (74.93, 24.257)
  arc A315 (74.549, 24.2189) -> (74.549, 24.2951) centre (74.549, 24.257) ccw
  arc A316 (74.93, 26.5049) -> (74.93, 26.5811) centre (74.93, 26.543) ccw
  line L157 (73.4314, 25.0952) -> (74.295, 25.0952)
  line L158 (74.295, 25.0952) -> (74.295, 25.7048)
  line L159 (81.5086, 25.7048) -> (80.645, 25.7048)
  arc A317 (75.057, 26.4541) -> (75.057, 26.3779) centre (75.057, 26.416) ccw
  line L160 (80.645, 24.511) -> (80.645, 26.289)
  arc A318 (79.9099, 24.4109) -> (79.8561, 24.3571) centre (79.883, 24.384) ccw
  arc A319 (80.391, 24.257) -> (80.645, 24.511) centre (80.391, 24.511) ccw
  arc A320 (79.8561, 26.4429) -> (79.9099, 26.3891) centre (79.883, 26.416) ccw
  arc A321 (80.391, 24.2189) -> (80.391, 24.2951) centre (80.391, 24.257) ccw
  arc A322 (74.549, 26.543) -> (74.295, 26.289) centre (74.549, 26.289) ccw
  arc A323 (60.3631, 21.209) -> (60.2869, 21.209) centre (60.325, 21.209) ccw
  arc A324 (79.883, 24.3459) -> (79.883, 24.4221) centre (79.883, 24.384) ccw
  arc A325 (79.883, 26.3779) -> (79.883, 26.4541) centre (79.883, 26.416) ccw
  arc A326 (75.057, 24.4221) -> (75.057, 24.3459) centre (75.057, 24.384) ccw
  arc A327 (74.549, 24.2951) -> (74.549, 24.2189) centre (74.549, 24.257) ccw
  arc A328 (74.295, 24.511) -> (74.549, 24.257) centre (74.549, 24.511) ccw
  arc A329 (74.3331, 24.511) -> (74.2569, 24.511) centre (74.295, 24.511) ccw
  line L161 (61.087, 21.336) -> (60.96, 21.463)
  line L162 (74.549, 26.543) -> (74.93, 26.543)
  line L163 (74.549, 24.257) -> (74.93, 24.257)
  line L164 (79.883, 24.384) -> (80.01, 24.257)
  line L165 (79.883, 26.416) -> (80.01, 26.543)
  arc A330 (80.6831, 24.511) -> (80.6069, 24.511) centre (80.645, 24.511) ccw
  arc A331 (80.645, 26.289) -> (80.391, 26.543) centre (80.391, 26.289) ccw
  line L166 (74.295, 25.7048) -> (73.4314, 25.7048)
  line L167 (79.883, 24.384) -> (75.057, 24.384)
  arc A332 (80.01, 26.5811) -> (80.01, 26.5049) centre (80.01, 26.543) ccw
  arc A333 (66.7131, 19.431) -> (66.6369, 19.431) centre (66.675, 19.431) ccw
  line L168 (80.645, 25.0952) -> (81.5086, 25.0952)
  line L169 (80.391, 24.257) -> (80.01, 24.257)
  line L170 (79.883, 26.416) -> (75.057, 26.416)
  arc A334 (74.2569, 26.289) -> (74.3331, 26.289) centre (74.295, 26.289) ccw
  arc A335 (74.9031, 24.2839) -> (74.9569, 24.2301) centre (74.93, 24.257) ccw
  arc A336 (80.01, 24.2951) -> (80.01, 24.2189) centre (80.01, 24.257) ccw
  line L171 (74.295, 24.511) -> (74.295, 26.289)
  arc A337 (74.549, 26.5049) -> (74.549, 26.5811) centre (74.549, 26.543) ccw
  arc A338 (80.6069, 24.511) -> (80.6831, 24.511) centre (80.645, 24.511) ccw
  line L172 (67.5386, 20.0152) -> (67.5386, 20.6248)
  arc A339 (61.0601, 21.3091) -> (61.1139, 21.3629) centre (61.087, 21.336) ccw
  arc A340 (60.579, 19.1389) -> (60.579, 19.2151) centre (60.579, 19.177) ccw
  line L173 (65.913, 21.336) -> (61.087, 21.336)
  line L174 (60.579, 21.463) -> (60.96, 21.463)
  arc A341 (60.579, 19.2151) -> (60.579, 19.1389) centre (60.579, 19.177) ccw
  arc A342 (60.579, 21.4249) -> (60.579, 21.5011) centre (60.579, 21.463) ccw
  line L175 (66.675, 20.0152) -> (67.5386, 20.0152)
  arc A343 (66.421, 19.177) -> (66.675, 19.431) centre (66.421, 19.431) ccw
  arc A344 (60.2869, 19.431) -> (60.3631, 19.431) centre (60.325, 19.431) ccw
  arc A345 (60.96, 21.4249) -> (60.96, 21.5011) centre (60.96, 21.463) ccw
  arc A346 (66.04, 19.2151) -> (66.04, 19.1389) centre (66.04, 19.177) ccw
  arc A347 (65.913, 19.2659) -> (65.913, 19.3421) centre (65.913, 19.304) ccw
  line L176 (66.421, 19.177) -> (66.04, 19.177)
  arc A348 (60.3631, 19.431) -> (60.2869, 19.431) centre (60.325, 19.431) ccw
  line L177 (59.4614, 20.6248) -> (59.4614, 20.0152)
  arc A349 (66.675, 21.209) -> (66.421, 21.463) centre (66.421, 21.209) ccw
  line L178 (65.913, 21.336) -> (66.04, 21.463)
  arc A350 (66.04, 21.5011) -> (66.04, 21.4249) centre (66.04, 21.463) ccw
  line L179 (60.325, 20.6248) -> (59.4614, 20.6248)
  arc A351 (66.421, 21.4249) -> (66.421, 21.5011) centre (66.421, 21.463) ccw
  arc A352 (60.325, 19.431) -> (60.579, 19.177) centre (60.579, 19.431) ccw
  arc A353 (60.3631, 24.511) -> (60.2869, 24.511) centre (60.325, 24.511) ccw
  line L180 (65.913, 26.416) -> (66.04, 26.543)
  arc A354 (61.087, 19.3421) -> (61.087, 19.2659) centre (61.087, 19.304) ccw
  line L181 (60.325, 19.431) -> (60.325, 21.209)
  arc A355 (66.421, 21.5011) -> (66.421, 21.4249) centre (66.421, 21.463) ccw
  line L182 (59.4614, 20.0152) -> (60.325, 20.0152)
  line L183 (65.913, 19.304) -> (61.087, 19.304)
  arc A356 (66.04, 24.2951) -> (66.04, 24.2189) centre (66.04, 24.257) ccw
  arc A357 (66.421, 26.5049) -> (66.421, 26.5811) centre (66.421, 26.543) ccw
  line L184 (60.325, 25.7048) -> (59.4614, 25.7048)
  arc A358 (66.0669, 26.5161) -> (66.0131, 26.5699) centre (66.04, 26.543) ccw
  arc A359 (66.7131, 21.209) -> (66.6369, 21.209) centre (66.675, 21.209) ccw
  line L185 (61.087, 19.304) -> (60.96, 19.177)
  line L186 (66.675, 20.6248) -> (66.675, 20.0152)
  arc A360 (65.913, 21.2979) -> (65.913, 21.3741) centre (65.913, 21.336) ccw
  arc A361 (66.6369, 21.209) -> (66.7131, 21.209) centre (66.675, 21.209) ccw
  arc A362 (61.1139, 19.2771) -> (61.0601, 19.3309) centre (61.087, 19.304) ccw
  arc A363 (60.579, 26.5049) -> (60.579, 26.5811) centre (60.579, 26.543) ccw
  arc A364 (60.579, 21.463) -> (60.325, 21.209) centre (60.579, 21.209) ccw
  arc A365 (66.0669, 21.4361) -> (66.0131, 21.4899) centre (66.04, 21.463) ccw
  line L187 (65.913, 24.384) -> (66.04, 24.257)
  arc A366 (66.7131, 24.511) -> (66.6369, 24.511) centre (66.675, 24.511) ccw
  line L188 (60.579, 19.177) -> (60.96, 19.177)
  line L189 (66.675, 19.431) -> (66.675, 21.209)
  arc A367 (66.6369, 19.431) -> (66.7131, 19.431) centre (66.675, 19.431) ccw
  arc A368 (61.087, 21.3741) -> (61.087, 21.2979) centre (61.087, 21.336) ccw
  line L190 (66.421, 21.463) -> (66.04, 21.463)
  arc A369 (65.8861, 21.3629) -> (65.9399, 21.3091) centre (65.913, 21.336) ccw
  arc A370 (66.421, 19.1389) -> (66.421, 19.2151) centre (66.421, 19.177) ccw
  line L191 (65.913, 19.304) -> (66.04, 19.177)
  arc A371 (66.421, 19.2151) -> (66.421, 19.1389) centre (66.421, 19.177) ccw
  arc A372 (60.9331, 19.2039) -> (60.9869, 19.1501) centre (60.96, 19.177) ccw
  line L192 (67.5386, 20.6248) -> (66.675, 20.6248)
  arc A373 (66.0131, 24.2301) -> (66.0669, 24.2839) centre (66.04, 24.257) ccw
  line L193 (66.421, 26.543) -> (66.04, 26.543)
  arc A374 (66.6369, 26.289) -> (66.7131, 26.289) centre (66.675, 26.289) ccw
  arc A375 (60.96, 19.1389) -> (60.96, 19.2151) centre (60.96, 19.177) ccw
  line L194 (60.325, 20.0152) -> (60.325, 20.6248)
  arc A376 (65.9399, 19.3309) -> (65.8861, 19.2771) centre (65.913, 19.304) ccw
  arc A377 (60.2869, 21.209) -> (60.3631, 21.209) centre (60.325, 21.209) ccw
  arc A378 (60.579, 21.5011) -> (60.579, 21.4249) centre (60.579, 21.463) ccw
  arc A379 (66.0131, 19.1501) -> (66.0669, 19.2039) centre (66.04, 19.177) ccw
  line L195 (67.5386, 25.0952) -> (67.5386, 25.7048)
  line L196 (59.4614, 25.0952) -> (60.325, 25.0952)
  arc A380 (42.799, 34.1249) -> (42.799, 34.2011) centre (42.799, 34.163) ccw
  arc A381 (60.9869, 26.5699) -> (60.9331, 26.5161) centre (60.96, 26.543) ccw
  line L197 (43.307, 34.036) -> (48.133, 34.036)
  arc A382 (42.799, 31.8389) -> (42.799, 31.9151) centre (42.799, 31.877) ccw
  arc A383 (48.641, 31.877) -> (48.895, 32.131) centre (48.641, 32.131) ccw
  arc A384 (60.579, 26.5811) -> (60.579, 26.5049) centre (60.579, 26.543) ccw
  arc A385 (43.1531, 31.9039) -> (43.2069, 31.8501) centre (43.18, 31.877) ccw
  arc A386 (66.7131, 26.289) -> (66.6369, 26.289) centre (66.675, 26.289) ccw
  line L198 (42.545, 33.909) -> (42.545, 32.131)
  arc A387 (42.5831, 33.909) -> (42.5069, 33.909) centre (42.545, 33.909) ccw
  arc A388 (60.579, 26.543) -> (60.325, 26.289) centre (60.579, 26.289) ccw
  arc A389 (60.96, 24.2189) -> (60.96, 24.2951) centre (60.96, 24.257) ccw
  arc A390 (60.3631, 26.289) -> (60.2869, 26.289) centre (60.325, 26.289) ccw
  arc A391 (65.9399, 24.4109) -> (65.8861, 24.3571) centre (65.913, 24.384) ccw
  line L199 (48.133, 32.004) -> (48.26, 31.877)
  line L200 (60.325, 26.289) -> (60.325, 24.511)
  line L201 (48.641, 31.877) -> (48.26, 31.877)
  arc A392 (60.96, 26.5049) -> (60.96, 26.5811) centre (60.96, 26.543) ccw
  line L202 (61.087, 26.416) -> (65.913, 26.416)
  line L203 (61.087, 26.416) -> (60.96, 26.543)
  arc A393 (60.2869, 24.511) -> (60.3631, 24.511) centre (60.325, 24.511) ccw
  arc A394 (60.579, 24.2189) -> (60.579, 24.2951) centre (60.579, 24.257) ccw
  arc A395 (61.1139, 24.3571) -> (61.0601, 24.4109) centre (61.087, 24.384) ccw
  arc A396 (48.895, 33.909) -> (48.641, 34.163) centre (48.641, 33.909) ccw
  arc A397 (42.799, 34.163) -> (42.545, 33.909) centre (42.799, 33.909) ccw
  line L204 (61.087, 24.384) -> (60.96, 24.257)
  line L205 (67.5386, 25.7048) -> (66.675, 25.7048)
  arc A398 (60.9331, 24.2839) -> (60.9869, 24.2301) centre (60.96, 24.257) ccw
  arc A399 (61.0601, 26.3891) -> (61.1139, 26.4429) centre (61.087, 26.416) ccw
  line L206 (60.325, 25.0952) -> (60.325, 25.7048)
  arc A400 (48.8569, 33.909) -> (48.9331, 33.909) centre (48.895, 33.909) ccw
  line L207 (59.4614, 25.7048) -> (59.4614, 25.0952)
  arc A401 (60.579, 24.2951) -> (60.579, 24.2189) centre (60.579, 24.257) ccw
  line L208 (60.579, 26.543) -> (60.96, 26.543)
  arc A402 (48.641, 34.2011) -> (48.641, 34.1249) centre (48.641, 34.163) ccw
  arc A403 (66.421, 26.5811) -> (66.421, 26.5049) centre (66.421, 26.543) ccw
  arc A404 (66.675, 26.289) -> (66.421, 26.543) centre (66.421, 26.289) ccw
  arc A405 (48.9331, 32.131) -> (48.8569, 32.131) centre (48.895, 32.131) ccw
  arc A406 (48.2869, 34.1361) -> (48.2331, 34.1899) centre (48.26, 34.163) ccw
  arc A407 (65.913, 24.3459) -> (65.913, 24.4221) centre (65.913, 24.384) ccw
  arc A408 (48.641, 31.9151) -> (48.641, 31.8389) centre (48.641, 31.877) ccw
  line L209 (42.545, 33.3248) -> (41.6814, 33.3248)
  arc A409 (60.2869, 26.289) -> (60.3631, 26.289) centre (60.325, 26.289) ccw
  arc A410 (66.421, 24.2951) -> (66.421, 24.2189) centre (66.421, 24.257) ccw
  line L210 (60.579, 24.257) -> (60.96, 24.257)
  line L211 (66.675, 25.0952) -> (67.5386, 25.0952)
  line L212 (43.307, 32.004) -> (48.133, 32.004)
  arc A411 (60.325, 24.511) -> (60.579, 24.257) centre (60.579, 24.511) ccw
  arc A412 (66.421, 24.2189) -> (66.421, 24.2951) centre (66.421, 24.257) ccw
  arc A413 (61.087, 26.4541) -> (61.087, 26.3779) centre (61.087, 26.416) ccw
  line L213 (61.087, 24.384) -> (65.913, 24.384)
  arc A414 (43.307, 34.0741) -> (43.307, 33.9979) centre (43.307, 34.036) ccw
  arc A415 (66.04, 26.5811) -> (66.04, 26.5049) centre (66.04, 26.543) ccw
  arc A416 (48.26, 31.9151) -> (48.26, 31.8389) centre (48.26, 31.877) ccw
  line L214 (66.421, 24.257) -> (66.04, 24.257)
  arc A417 (61.087, 24.4221) -> (61.087, 24.3459) centre (61.087, 24.384) ccw
  line L215 (66.675, 26.289) -> (66.675, 24.511)
  arc A418 (66.6369, 24.511) -> (66.7131, 24.511) centre (66.675, 24.511) ccw
  arc A419 (66.421, 24.257) -> (66.675, 24.511) centre (66.421, 24.511) ccw
  arc A420 (65.8861, 26.4429) -> (65.9399, 26.3891) centre (65.913, 26.416) ccw
  arc A421 (65.913, 26.3779) -> (65.913, 26.4541) centre (65.913, 26.416) ccw
  line L216 (66.675, 25.7048) -> (66.675, 25.0952)
  arc A422 (43.3339, 31.9771) -> (43.2801, 32.0309) centre (43.307, 32.004) ccw
  arc A423 (48.641, 31.8389) -> (48.641, 31.9151) centre (48.641, 31.877) ccw
  line L217 (49.7586, 38.4048) -> (48.895, 38.4048)
  line L218 (48.895, 33.909) -> (48.895, 32.131)
  arc A424 (48.9331, 33.909) -> (48.8569, 33.909) centre (48.895, 33.909) ccw
  line L219 (48.895, 38.4048) -> (48.895, 37.7952)
  arc A425 (48.1599, 37.1109) -> (48.1061, 37.0571) centre (48.133, 37.084) ccw
  line L220 (49.7586, 37.7952) -> (49.7586, 38.4048)
  arc A426 (48.641, 39.2049) -> (48.641, 39.2811) centre (48.641, 39.243) ccw
  arc A427 (48.26, 34.2011) -> (48.26, 34.1249) centre (48.26, 34.163) ccw
  line L221 (42.799, 39.243) -> (43.18, 39.243)
  line L222 (43.307, 37.084) -> (43.18, 36.957)
  line L223 (49.7586, 32.7152) -> (49.7586, 33.3248)
  arc A428 (48.1599, 32.0309) -> (48.1061, 31.9771) centre (48.133, 32.004) ccw
  arc A429 (42.5831, 38.989) -> (42.5069, 38.989) centre (42.545, 38.989) ccw
  arc A430 (48.2331, 31.8501) -> (48.2869, 31.9039) centre (48.26, 31.877) ccw
  line L224 (43.307, 39.116) -> (48.133, 39.116)
  arc A431 (43.307, 37.1221) -> (43.307, 37.0459) centre (43.307, 37.084) ccw
  arc A432 (42.5069, 38.989) -> (42.5831, 38.989) centre (42.545, 38.989) ccw
  line L225 (41.6814, 37.7952) -> (42.545, 37.7952)
  line L226 (48.895, 38.989) -> (48.895, 37.211)
  arc A433 (42.545, 37.211) -> (42.799, 36.957) centre (42.799, 37.211) ccw
  line L227 (42.545, 32.7152) -> (42.545, 33.3248)
  arc A434 (42.545, 32.131) -> (42.799, 31.877) centre (42.799, 32.131) ccw
  arc A435 (48.133, 33.9979) -> (48.133, 34.0741) centre (48.133, 34.036) ccw
  line L228 (48.895, 37.7952) -> (49.7586, 37.7952)
  arc A436 (48.8569, 32.131) -> (48.9331, 32.131) centre (48.895, 32.131) ccw
  arc A437 (42.799, 39.243) -> (42.545, 38.989) centre (42.799, 38.989) ccw
  arc A438 (48.1061, 34.0629) -> (48.1599, 34.0091) centre (48.133, 34.036) ccw
  arc A439 (48.8569, 37.211) -> (48.9331, 37.211) centre (48.895, 37.211) ccw
  arc A440 (42.5069, 37.211) -> (42.5831, 37.211) centre (42.545, 37.211) ccw
  line L229 (43.307, 37.084) -> (48.133, 37.084)
  arc A441 (48.8569, 38.989) -> (48.9331, 38.989) centre (48.895, 38.989) ccw
  arc A442 (43.307, 32.0421) -> (43.307, 31.9659) centre (43.307, 32.004) ccw
  arc A443 (48.133, 39.0779) -> (48.133, 39.1541) centre (48.133, 39.116) ccw
  line L230 (48.133, 39.116) -> (48.26, 39.243)
  line L231 (48.895, 32.7152) -> (49.7586, 32.7152)
  arc A444 (43.18, 31.8389) -> (43.18, 31.9151) centre (43.18, 31.877) ccw
  arc A445 (42.799, 31.9151) -> (42.799, 31.8389) centre (42.799, 31.877) ccw
  arc A446 (42.5069, 32.131) -> (42.5831, 32.131) centre (42.545, 32.131) ccw
  arc A447 (48.133, 31.9659) -> (48.133, 32.0421) centre (48.133, 32.004) ccw
  line L232 (48.133, 37.084) -> (48.26, 36.957)
  arc A448 (48.2869, 39.2161) -> (48.2331, 39.2699) centre (48.26, 39.243) ccw
  line L233 (42.799, 31.877) -> (43.18, 31.877)
  arc A449 (43.2069, 34.1899) -> (43.1531, 34.1361) centre (43.18, 34.163) ccw
  arc A450 (43.18, 34.1249) -> (43.18, 34.2011) centre (43.18, 34.163) ccw
  arc A451 (43.18, 36.9189) -> (43.18, 36.9951) centre (43.18, 36.957) ccw
  line L234 (48.641, 34.163) -> (48.26, 34.163)
  line L235 (42.799, 34.163) -> (43.18, 34.163)
  line L236 (43.307, 34.036) -> (43.18, 34.163)
  arc A452 (42.5831, 32.131) -> (42.5069, 32.131) centre (42.545, 32.131) ccw
  line L237 (48.133, 34.036) -> (48.26, 34.163)
  line L238 (49.7586, 33.3248) -> (48.895, 33.3248)
  arc A453 (43.2801, 34.0091) -> (43.3339, 34.0629) centre (43.307, 34.036) ccw
  line L239 (41.6814, 32.7152) -> (42.545, 32.7152)
  line L240 (43.307, 32.004) -> (43.18, 31.877)
  arc A454 (42.5069, 33.909) -> (42.5831, 33.909) centre (42.545, 33.909) ccw
  arc A455 (42.799, 34.2011) -> (42.799, 34.1249) centre (42.799, 34.163) ccw
  line L241 (41.6814, 33.3248) -> (41.6814, 32.7152)
  arc A456 (48.641, 34.1249) -> (48.641, 34.2011) centre (48.641, 34.163) ccw
  line L242 (42.545, 37.7952) -> (42.545, 38.4048)
  line L243 (48.895, 33.3248) -> (48.895, 32.7152)
  arc A457 (42.799, 39.2049) -> (42.799, 39.2811) centre (42.799, 39.243) ccw
  line L244 (48.641, 40.767) -> (48.26, 40.767)
  arc A458 (43.307, 40.9321) -> (43.307, 40.8559) centre (43.307, 40.894) ccw
  arc A459 (48.641, 39.2811) -> (48.641, 39.2049) centre (48.641, 39.243) ccw
  arc A460 (48.895, 42.799) -> (48.641, 43.053) centre (48.641, 42.799) ccw
  arc A461 (48.641, 36.9951) -> (48.641, 36.9189) centre (48.641, 36.957) ccw
  line L245 (48.641, 39.243) -> (48.26, 39.243)
  arc A462 (42.799, 36.9951) -> (42.799, 36.9189) centre (42.799, 36.957) ccw
  arc A463 (42.5831, 37.211) -> (42.5069, 37.211) centre (42.545, 37.211) ccw
  arc A464 (48.895, 38.989) -> (48.641, 39.243) centre (48.641, 38.989) ccw
  line L246 (42.545, 38.989) -> (42.545, 37.211)
  arc A465 (43.1531, 36.9839) -> (43.2069, 36.9301) centre (43.18, 36.957) ccw
  arc A466 (48.9331, 38.989) -> (48.8569, 38.989) centre (48.895, 38.989) ccw
  arc A467 (48.641, 36.957) -> (48.895, 37.211) centre (48.641, 37.211) ccw
  arc A468 (48.26, 39.2811) -> (48.26, 39.2049) centre (48.26, 39.243) ccw
  arc A469 (48.9331, 37.211) -> (48.8569, 37.211) centre (48.895, 37.211) ccw
  line L247 (48.641, 36.957) -> (48.26, 36.957)
  arc A470 (48.2331, 36.9301) -> (48.2869, 36.9839) centre (48.26, 36.957) ccw
  arc A471 (43.3339, 37.0571) -> (43.2801, 37.1109) centre (43.307, 37.084) ccw
  line L248 (43.307, 40.894) -> (43.18, 40.767)
  line L249 (41.6814, 38.4048) -> (41.6814, 37.7952)
  arc A472 (42.799, 39.2811) -> (42.799, 39.2049) centre (42.799, 39.243) ccw
  arc A473 (42.5069, 42.799) -> (42.5831, 42.799) centre (42.545, 42.799) ccw
  line L250 (48.895, 41.6052) -> (49.7586, 41.6052)
  arc A474 (42.799, 40.7289) -> (42.799, 40.8051) centre (42.799, 40.767) ccw
  line L251 (43.307, 39.116) -> (43.18, 39.243)
  arc A475 (43.18, 39.2049) -> (43.18, 39.2811) centre (43.18, 39.243) ccw
  arc A476 (42.799, 36.9189) -> (42.799, 36.9951) centre (42.799, 36.957) ccw
  line L252 (42.545, 41.021) -> (42.545, 42.799)
  line L253 (42.799, 36.957) -> (43.18, 36.957)
  arc A477 (48.8569, 42.799) -> (48.9331, 42.799) centre (48.895, 42.799) ccw
  line L254 (48.133, 42.926) -> (48.26, 43.053)
  line L255 (42.545, 38.4048) -> (41.6814, 38.4048)
  arc A478 (48.1061, 39.1429) -> (48.1599, 39.0891) centre (48.133, 39.116) ccw
  arc A479 (43.2801, 42.8991) -> (43.3339, 42.9529) centre (43.307, 42.926) ccw
  arc A480 (48.1599, 40.9209) -> (48.1061, 40.8671) centre (48.133, 40.894) ccw
  line L256 (48.895, 42.2148) -> (48.895, 41.6052)
  arc A481 (43.18, 40.7289) -> (43.18, 40.8051) centre (43.18, 40.767) ccw